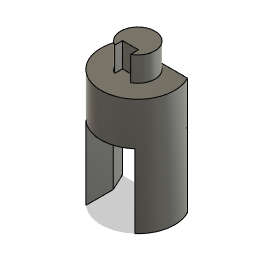
toolholder_wedge v3 (Autodesk Fusion 360 design; units mm, degrees)
Autodesk Fusion 360 part; units mm, degrees
sketch "Sketch1" plane through (0, 0, 0) normal (0, 1, 0) x (1, 0, 0)
  circle A0 centre (0, 0) radius 2.8
  circle A1 centre (0, 0) radius 6
  line L0 (0, 2.8) -> (5.3066, 2.8)
  line L1 (0, 2.8) -> (-5.3066, 2.8)
  line L2 (0, 0) -> (0, -1.2)
  line L3 (0, -1.2) -> (1.3, -1.2)
  line L4 (0, -1.2) -> (-1.3, -1.2)
  line L5 (-1.3, -1.2) -> (-1.3, -2.4799)
  line L6 (1.3, -1.2) -> (1.3, -2.4799)
  dimension "d1" = 5.6
  dimension "d2" = 12
  dimension "d22" = 1.2
  dimension "d23" = 1.3
  dimension "d24" = 1.3
  constraint coincident A0.centre A1.centre
  constraint coincident A0 L0.start
  constraint coincident A1 L0.end
  constraint tangent A0 L0
  constraint coincident A1 L1.end
  constraint tangent A0 L1
  constraint perpendicular L2 L3
  constraint perpendicular L2 L4
  constraint coincident A0 L5.end
  constraint perpendicular L4 L5
  constraint coincident A0 L6.end
  constraint perpendicular L3 L6
  measures "d1" diameter of A0
  measures "d2" diameter of A1
  measures "d22" distance of A0.centre L2.end
  measures "d23" distance of L2.end L3.end
  measures "d24" distance of L2.end L4.end
extrude "Extrude1" add sketch "Sketch1" along normal blind 6 contours A0 L3 L4 L5 L6 picked at (1.1387, -0.1888)
extrude "Extrude2" add sketch "Sketch1" along normal blind 2 contours A0 L3 L4 L5 L6 | A1 L0 L1 | A0 L3 L4 L5 L6 picked at (2.285, -4.3604)
extrude "Extrude3" add sketch "Sketch1" against normal blind 17 contours A0 L3 L4 L5 L6 | A1 L0 L1 | A0 L3 L4 L5 L6 picked at (2.285, -4.3604)
sketch "Sketch5" plane through (0, -17, 0) normal (0, -1, 0) x (1, 0, 0)
  line L0 (-5.3066, -2.8) -> (5.3066, -2.8)
  arc A0 (5.3066, -2.8) -> (-5.3066, -2.8) centre (0, 0) ccw
  line L1 (0, 0) -> (4, 0)
  line L2 (0, 0) -> (-4, 0)
  line L3 (-4, 0) -> (-4, 4.4721)
  line L4 (4, 0) -> (4, 4.4721)
  line L5 (4, 0) -> (5.3066, -2.8)
  line L6 (-4, 0) -> (-5.3066, -2.8)
  dimension "d39" = 4
  dimension "d40" = 4
  constraint coincident A0.centre L1.start
  constraint parallel L0 L1
  constraint parallel L1 L2
  constraint coincident A0 L3.end
  constraint perpendicular L2 L3
  constraint coincident A0 L4.end
  constraint perpendicular L1 L4
  constraint coincident L0.end A0.start
  constraint coincident L0.start A0.end
  measures "d39" distance of A0.centre L1.end
  measures "d40" distance of A0.centre L2.end
extrude "Extrude7" cut sketch "Sketch5" against normal blind 12 contours L0 L1 L2 L5 L6 | A0 L1 L2 L3 L4
